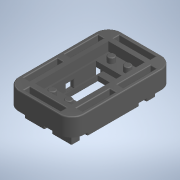
# Autodesk Inventor part: Main_v2
Saved by Autodesk Inventor 2020 (Build 240168000, 168)
## iProperties
Part Number: Main_v2
Material: Типовой
Document SubType Name: Обычные детали
Designer: User
Appearance: По умолчанию
Author: User
Autodesk Inventor part; units mm, degrees
ref_plane "Плоскость YZ" through (0, 0, 0) normal (1, 0, 0) x (0, 1, 0)
ref_plane "Плоскость XZ" through (0, 0, 0) normal (0, 1, 0) x (-1, 0, 0)
ref_plane "Плоскость XY" through (0, 0, 0) normal (0, 0, 1) x (1, 0, 0)
sketch "Главный" plane through (0, 0, 0) normal (0, 1, 0) x (-1, 0, 0)
  line L0 (-9.1667, -12.5) -> (9.1667, -12.5)
  line L1 (9.1667, -12.5) -> (9.1667, 12.5)
  line L2 (9.1667, 12.5) -> (-9.1667, 12.5)
  line L3 (-9.1667, 12.5) -> (-9.1667, -12.5)
  line L4 (-9.1667, -12.5) -> (9.1667, 12.5) construction
  line L5 (9.1667, -12.5) -> (-9.1667, 12.5) construction
  circle A0 centre (4.5833, -16.5) radius 1.9
  line L6 (0, 0) -> (9.1667, 0)
  line L7 (0, 0) -> (0, -12.5)
  circle A1 centre (4.5833, 16.5) radius 1.9
  circle A2 centre (-4.5833, -16.5) radius 1.9
  circle A3 centre (-4.5833, 16.5) radius 1.9
  line L8 (10.1667, 20.5) -> (-10.1667, 20.5)
  line L9 (-10.1667, 20.5) -> (-10.1667, -20.5)
  line L10 (-10.1667, -20.5) -> (10.1667, -20.5)
  line L11 (10.1667, -20.5) -> (10.1667, 20.5)
  line L12 (10.1667, 20.5) -> (-10.1667, -20.5) construction
  line L13 (-10.1667, 20.5) -> (10.1667, -20.5) construction
  line L14 (13.1667, 23.5) -> (-13.1667, 23.5)
  line L15 (-13.1667, 23.5) -> (-13.1667, -23.5)
  line L16 (-13.1667, -23.5) -> (13.1667, -23.5)
  line L17 (13.1667, -23.5) -> (13.1667, 23.5)
  line L18 (13.1667, 23.5) -> (-13.1667, -23.5) construction
  line L19 (-13.1667, 23.5) -> (13.1667, -23.5) construction
  line L20 (-18.2667, 28.6) -> (18.2667, 28.6)
  line L21 (18.2667, 28.6) -> (18.2667, -28.6)
  line L22 (18.2667, -28.6) -> (-18.2667, -28.6)
  line L23 (-18.2667, -28.6) -> (-18.2667, 28.6)
  line L24 (-18.2667, 28.6) -> (18.2667, -28.6) construction
  line L25 (18.2667, 28.6) -> (-18.2667, -28.6) construction
  line L26 (13.1667, -2.1) -> (16.2667, -2.1)
  line L27 (16.2667, -2.1) -> (16.2667, -20.7)
  line L28 (16.2667, -20.7) -> (13.1667, -20.7)
  line L29 (13.1667, 2.1) -> (16.2667, 2.1)
  line L30 (16.2667, 2.1) -> (16.2667, 20.7)
  line L31 (16.2667, 20.7) -> (13.1667, 20.7)
  line L32 (-13.1667, -2.1) -> (-16.2667, -2.1)
  line L33 (-16.2667, -2.1) -> (-16.2667, -20.7)
  line L34 (-16.2667, -20.7) -> (-13.1667, -20.7)
  line L35 (-13.1667, 2.1) -> (-16.2667, 2.1)
  line L36 (-16.2667, 2.1) -> (-16.2667, 20.7)
  line L37 (-16.2667, 20.7) -> (-13.1667, 20.7)
  line L38 (10.1667, -23.5) -> (10.1667, -26.6)
  line L39 (10.1667, -26.6) -> (-10.1667, -26.6)
  line L40 (-10.1667, -26.6) -> (-10.1667, -23.5)
  line L41 (10.1667, 23.5) -> (10.1667, 26.6)
  line L42 (10.1667, 26.6) -> (-10.1667, 26.6)
  line L43 (-10.1667, 26.6) -> (-10.1667, 23.5)
  point P0 (-13.1667, -20.7)
  point P1 (-13.1667, -2.1)
  point P2 (-13.1667, 2.1)
  point P3 (-13.1667, 20.7)
  point P4 (-10.1667, 23.5)
  point P5 (10.1667, 23.5)
  point P6 (13.1667, 20.7)
  point P7 (13.1667, 2.1)
  dimension "d0" = 18.3333
  dimension "d4" = 3.8
  dimension "d5" = 4
  dimension "d7" = 25
  dimension "d9" = 4.5833
  dimension "d10" = 1
  dimension "d11" = 4
  dimension "d12" = 3
  dimension "d13" = 3
  dimension "d28" = 3.1
  dimension "d31" = 18.6
  dimension "d32" = 4.2
  dimension "d33" = 2
  dimension "d34" = 3.1
  dimension "d35" = 20.3333
  dimension "d36" = 2
  constraints: 88 end point, 19 symmetric about line, 10 midpoint, 8 parallel, 7 perpendicular, 6 point on line, 5 horizontal, 4 centre point, 1 vertical, 3 other
  measures "d0" distance of L2.end L1.end
  measures "d4" diameter of A0
  measures "d5" distance from line of A0.centre L0
  measures "d7" distance between parallel lines of L0 L2
  measures "d9" distance from line of A0.centre L1
  measures "d10" distance between parallel lines of L1 L11
  measures "d11" distance from line of L10 A0.centre
  measures "d12" distance between parallel lines of L11 L17
  measures "d13" distance between parallel lines of L14 L8
  measures "d28" distance of L26.start L26.end
  measures "d31" distance of L26.end L27.end
  measures "d32" diameter of L26 L6
  measures "d33" distance between parallel lines of L27 L21
  measures "d34" distance of L38.start L38.end
  measures "d35" distance of L38.end L39.end
  measures "d36" distance between parallel lines of L22 L39
extrude "Пружина" add sketch "Главный" along normal blind 8 contours A0 | A1 | A2 | A3
extrude "Свобода" add sketch "Главный" along normal blind 5 contours L11 L10 L9 L8
extrude "Корпус" add sketch "Главный" along normal blind 10 contours L17 L16 L15 L14 | L20 L21 L22 L23
sketch "Для пластины" plane through (0, 0, 0) normal (0, -1, 0) x (1, 0, 0)
  line L0 (11.1667, 14.5) -> (-11.1667, 14.5)
  line L1 (-11.1667, 14.5) -> (-11.1667, -14.5)
  line L2 (-11.1667, -14.5) -> (11.1667, -14.5)
  line L3 (11.1667, -14.5) -> (11.1667, 14.5)
  line L4 (11.1667, 14.5) -> (-11.1667, -14.5) construction
  line L5 (-11.1667, 14.5) -> (11.1667, -14.5) construction
  point P0 (0, 0)
  dimension "d43" = 29
  dimension "d44" = 22.3333
  constraints: 12 end point, 2 midpoint, 2 parallel, 1 horizontal, 1 perpendicular
  measures "d43" distance between parallel lines of L2 L0
  measures "d44" distance between parallel lines of L1 L3
extrude "Пластина" cut sketch "Для пластины" against normal blind 3
sketch "Эскиз3" plane through (-10.1667, 0, 23.5) normal (0, 0, 1) x (1, 0, 0)
  line L0 (10.1667, 0) -> (10.1667, 5)
  line L1 (28.4333, 0) -> (-8.1, 0) projected
  line L2 (10.1667, 0) -> (28.4333, 0)
  line L3 (8.1667, 0) -> (8.1667, 5)
  line L4 (12.1667, 0) -> (12.1667, 5)
  line L5 (8.1667, 5) -> (12.1667, 5)
  dimension "d47" = 4
  dimension "d48" = 5
  constraints: 10 end point, 2 symmetric about line, 1 collinear, 1 midpoint, 1 perpendicular, 1 point on line, 1 vertical
  measures "d47" distance between parallel lines of L3 L4
  measures "d48" distance from line of L5 L0.start
extrude "Бок_Контроль_2" cut sketch "Эскиз3" against normal blind 2
mirror "Симетрия_бок_2" about plane through (0, 0, 0) normal (0, 0, 1) of "Бок_Контроль_2"
sketch "Эскиз4" plane through (-13.1667, 0, 2.1) normal (-1, 0, 0) x (0, 0, 1)
  line L0 (14.4, 0) -> (14.4, 10)
  line L1 (0, 10) -> (18.6, 10) projected
  line L2 (-16.6, 0) -> (12.4, 0) projected
  line L3 (12.4, 0) -> (12.4, 5)
  line L4 (16.4, 0) -> (16.4, 5)
  line L5 (12.4, 5) -> (16.4, 5)
  line L6 (10.4, 3) -> (10.4, 5) projected
  line L7 (18.6, 0) -> (0, 0) projected
  point P0 (-2.1, 0)
  dimension "d52" = 16.5
  dimension "d53" = 4
  dimension "d55" = 5
  constraints: 8 end point, 2 point on line, 2 symmetric about line, 2 vertical, 1 perpendicular
  measures "d52" distance from line of point (-2.1, 0) L0
  measures "d53" distance between parallel lines of L3 L4
  measures "d55" distance between parallel lines of L7 L5
extrude "Бок_Контроль_4" cut sketch "Эскиз4" against normal blind 2
mirror "Симетрия_бок_4_вертикаль" about plane through (0, 0, 0) normal (0, 0, 1) of "Бок_Контроль_4"
mirror "Симетрия_бок_4_горизонталь" about plane through (0, 0, 0) normal (1, 0, 0) of "Бок_Контроль_4", "Симетрия_бок_4_вертикаль"
sketch "Эскиз5" plane through (0, 0, 0) normal (0, -1, 0) x (1, 0, 0)
  line L0 (2, 21.5) -> (2, 23.5) projected
  line L1 (2, 23.5) -> (10.1667, 23.5) projected
  line L2 (10.1667, 23.5) -> (10.1667, 26.6) projected
  line L3 (10.1667, 26.6) -> (-10.1667, 26.6) projected
  line L4 (-10.1667, 26.6) -> (-10.1667, 23.5) projected
  line L5 (-10.1667, 23.5) -> (-2, 23.5) projected
  line L6 (-2, 23.5) -> (-2, 21.5) projected
  line L7 (-2, 21.5) -> (2, 21.5) projected
  line L8 (-16.2667, 2.1) -> (-13.1667, 2.1) projected
  line L9 (-13.1667, 2.1) -> (-13.1667, 14.5) projected
  line L10 (-13.1667, 14.5) -> (-11.1667, 14.5) projected
  line L11 (11.1667, 14.5) -> (-11.1667, 14.5) projected
  line L12 (11.1667, 14.5) -> (13.1667, 14.5) projected
  line L13 (13.1667, 14.5) -> (13.1667, 2.1) projected
  line L14 (13.1667, 2.1) -> (16.2667, 2.1) projected
  line L15 (16.2667, 2.1) -> (16.2667, 20.7) projected
  line L16 (16.2667, 20.7) -> (13.1667, 20.7) projected
  line L17 (13.1667, 20.7) -> (13.1667, 18.5) projected
  line L18 (13.1667, 18.5) -> (11.1667, 18.5) projected
  line L19 (11.1667, 18.5) -> (11.1667, 14.5) projected
  line L20 (-16.2667, 20.7) -> (-16.2667, 2.1) projected
  line L21 (-13.1667, 20.7) -> (-16.2667, 20.7) projected
  line L22 (-13.1667, 18.5) -> (-13.1667, 20.7) projected
  line L23 (-11.1667, 18.5) -> (-13.1667, 18.5) projected
  line L24 (-11.1667, 14.5) -> (-11.1667, 18.5) projected
  line L25 (-11.1667, 14.5) -> (-11.1667, -14.5) projected
  line L26 (-11.1667, -18.5) -> (-11.1667, -14.5) projected
  line L27 (-13.1667, -18.5) -> (-11.1667, -18.5) projected
  line L28 (-13.1667, -20.7) -> (-13.1667, -18.5) projected
  line L29 (-16.2667, -20.7) -> (-13.1667, -20.7) projected
  line L30 (-16.2667, -2.1) -> (-16.2667, -20.7) projected
  line L31 (-13.1667, -2.1) -> (-16.2667, -2.1) projected
  line L32 (-13.1667, -14.5) -> (-13.1667, -2.1) projected
  line L33 (-11.1667, -14.5) -> (-13.1667, -14.5) projected
  line L34 (-11.1667, -14.5) -> (11.1667, -14.5) projected
  line L35 (11.1667, -14.5) -> (11.1667, -18.5) projected
  line L36 (11.1667, -18.5) -> (13.1667, -18.5) projected
  line L37 (13.1667, -18.5) -> (13.1667, -20.7) projected
  line L38 (13.1667, -20.7) -> (16.2667, -20.7) projected
  line L39 (16.2667, -20.7) -> (16.2667, -2.1) projected
  line L40 (16.2667, -2.1) -> (13.1667, -2.1) projected
  line L41 (13.1667, -2.1) -> (13.1667, -14.5) projected
  line L42 (13.1667, -14.5) -> (11.1667, -14.5) projected
  line L43 (11.1667, -14.5) -> (11.1667, 14.5) projected
  line L44 (-10.1667, -26.6) -> (10.1667, -26.6) projected
  line L45 (10.1667, -26.6) -> (10.1667, -23.5) projected
  line L46 (10.1667, -23.5) -> (2, -23.5) projected
  line L47 (2, -23.5) -> (2, -21.5) projected
  line L48 (2, -21.5) -> (-2, -21.5) projected
  line L49 (-2, -21.5) -> (-2, -23.5) projected
  line L50 (-2, -23.5) -> (-10.1667, -23.5) projected
  line L51 (-10.1667, -23.5) -> (-10.1667, -26.6) projected
  line L52 (18.2667, 28.6) -> (18.2667, -28.6) projected
  line L53 (18.2667, -28.6) -> (-18.2667, -28.6) projected
  line L54 (-18.2667, -28.6) -> (-18.2667, 28.6) projected
  line L55 (-18.2667, 28.6) -> (18.2667, 28.6) projected
  line L56 (2, 23.5) -> (13.1667, 23.5)
  line L57 (13.1667, 23.5) -> (13.1667, 18.5)
  line L58 (11.1667, 18.5) -> (11.1667, 21.5)
  line L59 (11.1667, 21.5) -> (2, 21.5)
  line L60 (13.1667, 2.1) -> (11.1667, 2.1)
  line L61 (11.1667, 14.5) -> (11.1667, -14.5) projected
  line L62 (13.1667, -2.1) -> (11.1667, -2.1)
  line L63 (-13.1667, -2.1) -> (-11.1667, -2.1)
  line L64 (-11.1667, -14.5) -> (-11.1667, 14.5) projected
  line L65 (-13.1667, 2.1) -> (-11.1667, 2.1)
  line L66 (13.1667, -20.7) -> (13.1667, -23.5)
  line L67 (13.1667, -23.5) -> (11.1667, -23.5)
  line L68 (11.1667, -14.5) -> (11.1667, -18.5) projected
  line L69 (11.1667, -23.5) -> (11.1667, -18.5)
  line L70 (-2, -21.5) -> (2, -21.5) projected
  line L71 (11.1667, 0) -> (-11.1667, 0)
  line L72 (11.1667, -14.5) -> (-11.1667, -14.5) projected
  line L73 (0, -14.5) -> (0, 14.5)
  line L74 (-2, 23.5) -> (-13.1667, 23.5)
  line L75 (-13.1667, 23.5) -> (-13.1667, 18.5)
  line L76 (-11.1667, 18.5) -> (-11.1667, 21.5)
  line L77 (-11.1667, 21.5) -> (-2, 21.5)
  line L78 (-13.1667, -20.7) -> (-13.1667, -23.5)
  line L79 (-13.1667, -23.5) -> (-11.1667, -23.5)
  line L80 (-11.1667, -23.5) -> (-11.1667, -18.5)
  point P0 (-10.1667, 23.5)
  point P1 (-13.1667, 20.7)
  dimension "d74" = 5
  constraints: 40 end point, 6 point on line, 4 midpoint, 4 symmetric about line, 3 perpendicular, 2 parallel, 2 vertical, 1 collinear, 1 horizontal
  measures "d74" distance between parallel lines of L36 L67
extrude "Стенка_КонтрольПластина" add sketch "Эскиз5" along normal blind 6.6 contours L0 L1 L56 L57 L17 L18 L58 L59 | L77 L76 L23 L22 L75 L74 L5 L6 | L12 L13 L60 L43 | L25 L65 L9 L10 | L62 L41 L42 L43 | L25 L33 L32 L63 | L80 L79 L78 L28 L27 | L36 L37 L66 L67 L69
sketch "Эскиз6" plane through (11.1667, 0, 18.5) normal (-1, 0, 0) x (0, 0, 1)
  line L0 (3, -6.6) -> (0, -6.6) projected
  line L1 (-4, 5) -> (-4, -6.6) projected
  line L2 (3, -6.6) -> (-4, -6.6)
  line L3 (-4, -6.6) -> (-4, -3.6)
  line L4 (-4, -3.6) -> (3, -3.6)
  line L5 (3, -3.6) -> (3, -6.6)
  line L6 (-33, 5) -> (-33, -6.6) projected
  line L7 (-42, 0) -> (-42, -6.6) projected
  line L8 (-33, -6.6) -> (-42, -6.6)
  line L9 (-42, -6.6) -> (-42, -3.6)
  line L10 (-42, -3.6) -> (-33, -3.6)
  line L11 (-33, -3.6) -> (-33, -6.6)
  point P0 (-18.5, 0)
  dimension "d77" = 3
  dimension "d78" = 3
  constraints: 16 end point, 4 parallel, 2 horizontal, 2 perpendicular, 2 point on line
  measures "d77" distance between parallel lines of L2 L4
  measures "d78" distance between parallel lines of L10 L8
extrude "Задний_зажим_пластины" add sketch "Эскиз6" along normal blind 22.3333
sketch "Эскиз7" plane through (-11.1667, 0, 14.5) normal (1, 0, 0) x (0, 0, -1)
  line L0 (0, 5) -> (0, -6.6) projected
  line L1 (29, -6.6) -> (0, -6.6)
  line L2 (0, -6.6) -> (0, -3.6)
  line L3 (0, -3.6) -> (29, -3.6)
  line L4 (29, -3.6) -> (29, -6.6)
  point P0 (14.5, 0)
  point P1 (0, -6.6)
  dimension "d81" = 3
  constraints: 8 end point, 2 parallel, 1 horizontal, 1 perpendicular, 1 point on line
  measures "d81" distance between parallel lines of L3 L1
extrude "Боковой_зажим_пластины" add sketch "Эскиз7" along normal blind 1
mirror "Симетрия_боковой_контроль" about plane through (0, 0, 0) normal (1, 0, 0) of "Боковой_зажим_пластины"
sketch "Эскиз8" plane through (11.1667, -3.6, -14.5) normal (0, 1, 0) x (1, 0, 0)
  line L0 (-9.1667, 9) -> (-13.1667, 9) projected
  line L1 (-9.1667, 9) -> (-9.1667, 7) projected
  line L2 (-13.1667, 7) -> (-9.1667, 7) projected
  line L3 (-13.1667, 9) -> (-13.1667, 7) projected
  point P0 (-11.1667, -14.5)
extrude "Выдавливание10" cut sketch "Эскиз8" against normal blind 3
fillet "Сопряжение1" radius 7 4 edges at (18.2667, 5, 28.6) (18.2667, 5, -28.6) (-18.2667, 5, 28.6) (-18.2667, 5, -28.6)
fillet "Сопряжение2" radius 0.5 42 edges at (-13.1667, 10, -11.4) (-16.2667, 10, -11.4) (-14.7167, 10, -20.7) (-14.7167, 10, -2.1) (-14.7167, 10, 2.1) (-16.2667, 10, 11.4) (-13.1667, 10, 11.4) (-14.7167, 10, 20.7) (0, 10, 23.5) (-10.1667, 10, 25.05) (0, 10, 26.6) (10.1667, 10, 25.05) (14.7167, 10, 20.7) (16.2667, 10, 11.4) (13.1667, 10, 11.4) (14.7167, 10, 2.1) (14.7167, 10, -2.1) (13.1667, 10, -11.4) (16.2667, 10, -11.4) (14.7167, 10, -20.7) (0, 10, -23.5) (0, 10, -26.6) (-10.1667, 10, -25.05) (10.1667, 10, -25.05) (-16.2667, 0, 11.4) (-14.7167, 0, 20.7) (-10.1667, 0, 25.05) (0, 0, 26.6) (10.1667, 0, 25.05) (14.7167, 0, 20.7) (16.2667, 0, 11.4) (14.7167, 0, -2.1) (16.2667, 0, -11.4) (14.7167, 0, -20.7) (-14.7167, 0, 2.1) (14.7167, 0, 2.1) (-14.7167, 0, -2.1) (-16.2667, 0, -11.4) (-14.7167, 0, -20.7) (0, 0, -26.6) (-10.1667, 0, -25.05) (10.1667, 0, -25.05)
fillet "Сопряжение3" radius 0.5 4 edges at (-2.6833, 8, 16.5) (6.4833, 8, 16.5) (-2.6833, 8, -16.5) (6.4833, 8, -16.5)
fillet "Сопряжение4" radius 0.5 22 edges at (0, 0, -21.5) (2, 0, -22.5) (2, -3.6, -22.5) (0, -3.6, -21.5) (-2, 0, -22.5) (-2, -3.6, -22.5) (10.4167, 0, -23.5) (6.0833, 0, -23.5) (-10.4167, 0, -23.5) (-6.0833, 0, -23.5) (-6.5833, -3.6, -23.5) (6.5833, -3.6, -23.5) (11.1667, -1.8, -23.5) (-11.1667, -1.8, -23.5) (-11.1667, -3.6, -16.5) (-11.1667, -3.6, 16.5) (0, 0, 21.5) (0, -3.6, 21.5) (11.1667, -3.6, 16.5) (11.1667, -3.6, -16.5) (11.1667, -3.6, 0) (-11.1667, -3.6, 0)
fillet "Сопряжение5" radius 0.5 6 edges at (-11.1667, 0, 0) (-11.1667, -1.8, 2.1) (-11.1667, -1.8, -2.1) (11.1667, 0, 0) (11.1667, -1.8, 2.1) (11.1667, -1.8, -2.1)
fillet "Сопряжение7" radius 0.5 4 edges at (13.1667, -3.3, -23.5) (-13.1667, -3.3, -23.5) (-13.1667, -3.3, 23.5) (13.1667, -3.3, 23.5)
fillet "Сопряжение8" radius 0.5 4 edges at (0, -6.6, 14.5) (10.1667, -6.6, 0) (-10.1667, -6.6, 0) (0, -6.6, -14.5)
sketch "Эскиз9" plane through (-11.1667, 0, 14.5) normal (-1, 0, 0) x (0, 0, 1)
  line L0 (-12.4, -4.1) -> (-16.6, -4.1) projected
  line L1 (-16.6, 0) -> (-16.6, -6.6) projected
  line L2 (-12.4, -4.1) -> (-16.6, -4.1)
  line L3 (-16.6, -4.1) -> (-16.6, -6.6)
  line L4 (-16.6, -6.6) -> (-12.4, -6.6)
  line L5 (-12.4, -6.6) -> (-12.4, -4.1)
  point P0 (-14.5, 0)
  constraints: 8 end point, 2 parallel, 1 horizontal, 1 perpendicular
extrude "Выдавливание11" add sketch "Эскиз9" along normal blind 2
mirror "Зеркальное отражение5" about plane through (0, 0, 0) normal (1, 0, 0) of "Выдавливание11"
fillet "Сопряжение10" radius 0.6 26 edges at (-13.1667, -0.8, -14.5) (-13.1667, -0.8, -18.5) (-13.1667, -0.8, 18.5) (-13.1667, -0.8, 14.5) (13.1667, -0.8, -14.5) (13.1667, -0.8, -18.5) (13.1667, 5, -16.5) (13.1667, -0.8, 18.5) (13.1667, 5, 16.5) (13.1667, -0.8, 14.5) (-2.1464, 0.1464, -23.3536) (-2, 2.75, -23.5) (2.1464, 0.1464, -23.3536) (2, 2.75, -23.5) (0, 5, -23.5) (-2, -0.8, 23.5) (2, -0.8, 23.5) (0, 5, 23.5) (-18.2667, 10, 0) (-16.2164, 10, -26.5497) (0, 10, -28.6) (16.2164, 10, -26.5497) (18.2667, 10, 0) (16.2164, 10, 26.5497) (0, 10, 28.6) (-16.2164, 10, 26.5497)
equation "\"d9\" = 0.25 * d0"
equation "\"d13\" = d12"
equation "\"d28\" = d34"
equation "\"d35\" = d0 + 2 * d10"
equation "\"d36\" = d33"
equation "\"d52\" = 0.5 * d7 + d5"
equation "\"d53\" = d47"
equation "\"d55\" = d48"
equation "\"d74\" = d12 + d5 + 0.5 * d7 + d11 - 0.5 * d53 - d52"
equation "\"d78\" = d77"
